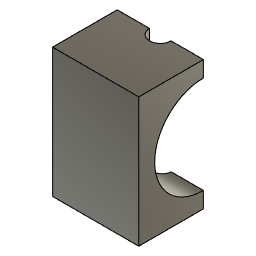
Cross Strut Holes v2 (Autodesk Fusion 360 design; units mm, degrees)
Autodesk Fusion 360 part; units mm, degrees
sketch "Sketch1" plane through (0, 0, 0) normal (1, 0, 0) x (0, 1, 0)
  line L0 (19.05, 38.1) -> (0, 38.1)
  line L1 (0, 38.1) -> (0, 0)
  line L2 (0, 0) -> (19.05, 0)
  line L3 (19.05, 0) -> (19.05, 4.699)
  line L4 (19.05, 38.1) -> (19.05, 33.401)
  line L5 (19.05, 33.401) -> (19.05, 4.699) construction
  arc A0 (19.05, 33.401) -> (19.05, 4.699) centre (19.05, 19.05) ccw
  dimension "d1" = 14.351
  dimension "d3" = 19.05
  dimension "d4" = 38.1
  constraint horizontal L0
  constraint coincident L1.end L2.start
  constraint parallel L0 L2
  constraint perpendicular L2 L3
  constraint perpendicular L0 L4
  constraint vertical L5
  constraint vertical L1
  constraint equal L3 L4
  constraint coincident L5 A0.centre
  measures "d1" radius of A0
  measures "d3" distance of L1 A0.centre
  measures "d4" distance of L0.end L1.end
extrude "Extrude1" add sketch "Sketch1" along normal blind 25.4
sketch "Sketch2" plane through (0, 0, 38.1) normal (0, 0, 1) x (-1, 0, 0)
  line L0 (0, -19.05) -> (0, 0)
  line L1 (0, 0) -> (-25.4, 0)
  line L2 (-25.4, 0) -> (-25.4, -19.05)
  line L3 (-25.4, -19.05) -> (0, -19.05)
  circle A0 centre (-12.7, -19.05) radius 3.175
  dimension "d7" = 6.35
  constraint midpoint L3 A0.centre
  measures "d7" diameter of A0
extrude "Extrude2" cut sketch "Sketch2" against normal up to surface (38.1 mm away) contours L3 A0 | L3 A0
